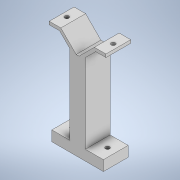
# Autodesk Inventor part: Fan_bottom
Saved by Autodesk Inventor 2022 (Build 260153000, 153)
## iProperties
Created: 2022-04-06
Part Number: Fan_bottom
Material: Generic
Document SubType Name: Modeling
Designer: Dani
Density: 1 g/cm^3
Appearance: Default
Author: Dani
## iProperties of the stored document Fan_bottom_3DPrint.ipt
Created: 2022-04-06
Part Number: Fan_bottom_3DPrint
Material: Generic
Document SubType Name: Modeling
Designer: Dani
Density: 1 g/cm^3
Appearance: Default
Author: Dani
Autodesk Inventor part; units mm, degrees
ref_plane "YZ Plane" through (0, 0, 0) normal (1, 0, 0) x (0, 1, 0)
ref_plane "XZ Plane" through (0, 0, 0) normal (0, 1, 0) x (-1, 0, 0)
ref_plane "XY Plane" through (0, 0, 0) normal (0, 0, 1) x (1, 0, 0)
sketch "Sketch1" plane through (0, 0, 0) normal (0, 0, 1) x (1, 0, 0)
  line L0 (0, -124.1012) -> (0, 44.6073) projected
  line L1 (0, 44.6073) -> (0, -124.1012) projected
  line L2 (-38.5085, 0) -> (38.5085, 0) projected
  line L3 (0, -16.2635) -> (16.2635, 0)
  line L4 (16.2635, 0) -> (0, 16.2635)
  line L5 (0, 16.2635) -> (-16.2635, 0)
  line L6 (-16.2635, 0) -> (0, -16.2635)
  line L7 (0, -16.2635) -> (0, 16.2635) construction
  line L8 (16.2635, 0) -> (-16.2635, 0) construction
  line L9 (0, -16.2635) -> (23, -16.2635) construction
  line L10 (0, -20.5061) -> (-17.5061, -3)
  line L11 (-17.5061, -3) -> (-27.5061, -3)
  line L12 (-27.5061, -3) -> (-27.5061, 3)
  line L13 (-27.5061, 3) -> (-17.5061, 3)
  line L14 (-17.5061, 3) -> (0, 20.5061)
  line L15 (0, 20.5061) -> (17.5061, 3)
  line L16 (17.5061, -3) -> (0, -20.5061)
  line L17 (-38.5085, 0) -> (38.5085, 0) projected
  line L18 (-27.5061, 0) -> (-16.2635, 0)
  line L19 (16.2635, 0) -> (23.5061, 0)
  line L20 (17.5061, -3) -> (27.5061, -3)
  line L21 (27.5061, -3) -> (27.5061, 3)
  line L22 (27.5061, 3) -> (17.5061, 3)
  line L23 (16.2635, 0) -> (27.5061, 0)
  line L24 (-7.5, -13.0061) -> (-7.5, -90)
  line L25 (-7.5, -90) -> (-25, -90)
  line L26 (-25, -90) -> (-25, -100)
  line L27 (-25, -100) -> (25, -100)
  line L28 (25, -100) -> (25, -90)
  line L29 (25, -90) -> (7.5, -90)
  line L30 (7.5, -90) -> (7.5, -13.0061)
  point P0 (0, 0)
  point P1 (-16.2635, 0)
  point P2 (16.2635, 0)
  point P3 (27.5061, 0)
  point P4 (16.2635, 0)
  point P5 (-16.2635, 0)
  dimension "d34" = 23
  dimension "d35" = 45
  dimension "d36" = 23
  dimension "d37" = 3
  dimension "d38" = 3
  dimension "d39" = 45
  dimension "d41" = 6
  dimension "d49" = 10
  dimension "d50" = 6
  dimension "d51" = 3
  dimension "d52" = 10
  dimension "d69" = 15
  dimension "d70" = 50
  dimension "d71" = 10
  dimension "d72" = 100
  constraints: 54 end point, 11 perpendicular, 7 point on line, 5 midpoint, 3 horizontal, 3 parallel, 1 equal length, 1 vertical, 5 other
  measures "d34" distance of L3.start L3.end
  measures "d35" angle of L9 L3
  measures "d36" distance of L4.end L3.end
  measures "d37" distance between parallel lines of L10 L6
  measures "d38" distance between parallel lines of L14 L5
  measures "d39" angle of L0 L16
  measures "d41" distance between parallel lines of L13 L11
  measures "d49" distance from line of L12 L13.end
  measures "d50" distance between parallel lines of L20 L22
  measures "d51" distance between parallel lines of L20 L2
  measures "d52" distance of L21.end L15.end
  measures "d69" distance between parallel lines of L30 L24
  measures "d70" distance between parallel lines of L28 L26
  measures "d71" distance between parallel lines of L27 L29
  measures "d72" distance between parallel lines of L27 L2
extrude "Extrusion3" add sketch "Sketch1" along normal blind 24 contours L10 L11 L12 L2 L6 L0 | L16 L30 L29 L28 L27 L0 | L0 L27 L26 L25 L24 L10 | L0 L3 L2 L21 L20 L16
sketch "Sketch4" plane through (-27.5061, 0, 0) normal (0, 1, 0) x (1, 0, 0)
  line L0 (11.2426, 0) -> (0, 0) projected
  line L1 (55.0122, 0) -> (43.7696, 0) projected
  line L2 (0, 0) -> (0, -24) projected
  line L3 (55.0122, 0) -> (55.0122, -24) projected
  point P0 (27.5061, 0)
  point P1 (5, -12)
  point P2 (50.0122, -12)
  dimension "d75" = 12
  dimension "d76" = 12
  dimension "d77" = 5
  dimension "d78" = 5
  measures "d75" distance from line of L0 point (5, -12)
  measures "d76" distance from line of L1 point (50.012, -12)
  measures "d77" distance from line of L2 point (5, -12)
  measures "d78" distance from line of point (50.012, -12) L3
hole "Hole2" at (-22.5061, 0, 12) at (22.5061, 0, 12) direction (0, -1, 0) diameter 4 depth 3
chamfer "Chamfer2" distance 2 angle 45 1 edges at (0, -16.2635, 12)
sketch "Sketch5" plane through (-25, -100, 0) normal (0, -1, 0) x (1, 0, 0)
  line L0 (-2.5061, 0) -> (-2.5061, 24) projected
  line L1 (52.5061, 0) -> (52.5061, 24) projected
  line L2 (0, 24) -> (50, 24) projected
  line L3 (0, 0) -> (0, 24) projected
  line L4 (50, 0) -> (50, 24) projected
  point P0 (25, 0)
  point P1 (8, 12)
  point P2 (42, 12)
  dimension "d91" = 12
  dimension "d92" = 12
  dimension "d93" = 8
  dimension "d94" = 8
  measures "d91" distance from line of L2 point (8, 12)
  measures "d92" distance from line of L2 point (42, 12)
  measures "d93" distance from line of L3 point (8, 12)
  measures "d94" distance from line of L4 point (42, 12)
hole "Hole3" at (-17, -100, 12) at (17, -100, 12) direction (0, 1, 0) diameter 4 depth 10
body "Solid3"
